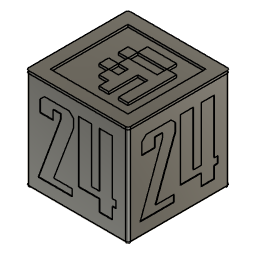
AutonOhm Apriltag 24 (Autodesk Fusion 360 design; units mm, degrees)
Autodesk Fusion 360 part; units mm, degrees
sketch "Skizze1" plane through (0, 0, 0) normal (0, 0, 1) x (1, 0, 0)
  line L0 (21, -21) -> (-21, -21)
  line L1 (-21, -21) -> (-21, 21)
  line L2 (-21, 21) -> (21, 21)
  line L3 (21, 21) -> (21, -21)
  line L4 (21, -21) -> (-21, 21) construction
  line L5 (-21, -21) -> (21, 21) construction
  dimension "d1" = 42
  dimension "d2" = 42
  constraint horizontal L0
  constraint perpendicular L0 L1
  constraint parallel L0 L2
  constraint parallel L1 L3
  constraint coincident L4 origin
  constraint coincident L5 origin
  measures "d1" distance of L1.end L2.end
  measures "d2" distance of L0.end L1.end
extrude "Extrusion1" add sketch "Skizze1" along normal blind 41 makes body 1
sketch "Skizze2" plane through (0, 0, 41) normal (0, 0, 1) x (-1, 0, 0)
  line L0 (-21, -21) -> (21, -21)
  line L1 (21, -21) -> (21, 21)
  line L2 (21, 21) -> (-21, 21)
  line L3 (-21, 21) -> (-21, -21)
  line L4 (21, -21) -> (-21, -21)
  line L5 (-21, -21) -> (-21, 21)
  line L6 (-21, 21) -> (21, 21)
  line L7 (21, 21) -> (21, -21)
  line L8 (-16, 16) -> (16, 16)
  line L9 (16, 16) -> (16, -16)
  line L10 (16, -16) -> (-16, -16)
  line L11 (-16, -16) -> (-16, 16)
  line L12 (-16, 16) -> (16, -16) construction
  line L13 (16, 16) -> (-16, -16) construction
  dimension "d5" = 32
  dimension "d6" = 32
  constraint horizontal L4
  constraint vertical L5
  constraint horizontal L6
  constraint vertical L7
  constraint coincident L2.end L3.start
  constraint coincident L0.end L1.start
  constraint horizontal L8
  constraint perpendicular L8 L9
  constraint parallel L8 L10
  constraint parallel L9 L11
  constraint coincident L12 origin
  constraint coincident L13 origin
  measures "d5" distance of L9.end L10.end
  measures "d6" distance of L8.end L9.end
extrude "Extrusion2" add sketch "Skizze2" along normal blind 1 separate body makes body 2
fillet "Abrundung1" radius 1 8 edges at (-21, 21, 20.5) (-21, -21, 20.5) (-21, 0, 0) (0, -21, 0) (21, -21, 20.5) (21, 0, 0) (21, 21, 20.5) (0, 21, 0) on bodies 1
fillet "Abrundung2" radius 1 1 edges at (21, 21, 41.5) on bodies 2
fillet "Abrundung3" radius 1 1 edges at (21, -21, 41.5) on bodies 2
fillet "Abrundung4" radius 1 1 edges at (-21, -21, 41.5) on bodies 2
fillet "Abrundung5" radius 1 1 edges at (-21, 21, 41.5) on bodies 2
sketch "Skizze3" plane through (0, 0, 0) normal (0, 0, -1) x (1, 0, 0)
  line L0 (-20, -20) -> (20, -20)
  line L1 (20, -20) -> (20, 20)
  line L2 (20, 20) -> (-20, 20)
  line L3 (-20, 20) -> (-20, -20)
  line L4 (-15.5554, -7.5319) -> (-15.5554, -12.9394)
  line L5 (-15.5554, -12.9394) -> (-1.7653, -13.0619)
  line L6 (-1.7653, -13.0619) -> (-1.8353, -7.8468)
  spline S0 degree 3 poles (-1.8353, -7.8468) (-9.4573, -5.9337) (-9.4543, 8.1703) (-0.2245, 8.2733) knots 0 0 0 0 1 1 1 1
  spline S1 degree 3 poles (-0.2245, 8.2733) (9.1628, 8.378) (10.5465, -5.8261) (1.9583, -7.8813) knots 0 0 0 0 1 1 1 1
  line L7 (1.9583, -7.8813) -> (1.9723, -13.0334)
  spline S2 degree 3 poles (1.9723, -13.0334) (15.5516, -12.9722) (18.9797, 12.8679) (-0.1523, 13.061) knots 0 0 0 0 1 1 1 1
  spline S3 degree 3 poles (-0.1523, 13.061) (-11.1806, 13.1724) (-15.9327, 2.2058) (-10.2013, -7.6521) knots 0 0 0 0 1 1 1 1
  line L8 (-10.2013, -7.6521) -> (-15.5554, -7.5319)
extrude "Extrusion3" add sketch "Skizze3" against normal blind 0.6 separate body contours L4 L5 L6 S0 S1 L7 S2 S3 L8 makes body 3
sketch "Skizze4" plane through (0, 0, 41) normal (0, 0, 1) x (-1, 0, 0)
  arc A0 (21, 20) -> (20, 21) centre (20, 20) ccw
  line L0 (20, 21) -> (-20, 21)
  arc A1 (-20, 21) -> (-21, 20) centre (-20, 20) ccw
  line L1 (-21, 20) -> (-21, -20)
  arc A2 (-21, -20) -> (-20, -21) centre (-20, -20) ccw
  line L2 (-20, -21) -> (20, -21)
  arc A3 (20, -21) -> (21, -20) centre (20, -20) ccw
  line L3 (21, -20) -> (21, 20)
  line L4 (-19.9999, 19.9999) -> (20.0001, 19.9999)
  line L5 (20.0001, 19.9999) -> (20.0001, -20.0001)
  line L6 (20.0001, -20.0001) -> (-19.9999, -20.0001)
  line L7 (-19.9999, -20.0001) -> (-19.9999, 19.9999)
  line L8 (21, 21) -> (-21, 21)
  line L9 (-21, 21) -> (-21, -21)
  line L10 (-21, -21) -> (21, -21)
  line L11 (21, -21) -> (21, 21)
  line L12 (20.0001, 19.9999) -> (-19.9999, 19.9999)
  line L13 (-19.9999, 19.9999) -> (-19.9999, -20.0001)
  line L14 (-19.9999, -20.0001) -> (20.0001, -20.0001)
  line L15 (20.0001, -20.0001) -> (20.0001, 19.9999)
  line L16 (-12.038, 11.9999) -> (-12.038, -7.9999)
  line L17 (-12.038, -7.9999) -> (-8.0381, -7.9999)
  line L18 (-8.0381, -7.9999) -> (-8.0381, -11.9999)
  line L19 (-8.0381, -11.9999) -> (3.9619, -11.9999)
  line L20 (3.9619, -11.9999) -> (3.9619, -7.9999)
  line L21 (3.9619, -7.9999) -> (7.9621, -7.9999)
  line L22 (7.9621, -7.9999) -> (7.9621, -4)
  line L23 (7.9621, -4) -> (3.9619, -4)
  line L24 (3.9619, -4) -> (3.9619, 0)
  line L25 (3.9619, 0) -> (7.9621, 0)
  line L26 (7.9621, 0) -> (7.9621, 4)
  line L27 (7.9621, 4) -> (3.9619, 4)
  line L28 (3.9619, 4) -> (3.9619, 8)
  line L29 (3.9619, 8) -> (-0.0381, 8)
  line L30 (-0.0381, 8) -> (-0.0381, 11.9999)
  line L31 (-0.0381, 11.9999) -> (-4.0381, 11.9999)
  line L32 (-4.0381, 11.9999) -> (-4.0381, 0)
  line L33 (-4.0381, 0) -> (-8.0381, 0)
  line L34 (-8.0381, 0) -> (-8.0381, 11.9999)
  line L35 (-8.0381, 11.9999) -> (-12.038, 11.9999)
  line L36 (-0.0381, 4) -> (-0.0381, 0)
  line L37 (-0.0381, 0) -> (3.9619, 0)
  line L38 (3.9619, 0) -> (3.9619, 4)
  line L39 (3.9619, 4) -> (-0.0381, 4)
  line L40 (-8.0381, -3.9999) -> (-8.0381, -7.9999)
  line L41 (-8.0381, -7.9999) -> (3.9619, -7.9999)
  line L42 (3.9619, -7.9999) -> (3.9619, -4)
  line L43 (3.9619, -4) -> (-8.0381, -3.9999)
extrude "Extrusion4" add sketch "Skizze4" along normal blind 1 separate body contours L16 L17 L24 L28 L29 L30 L31 L32 L33 L34 L35 L36 L37 L39 L40 L43 | L18 L19 L20 L41 | L21 L22 L23 L42 | L25 L26 L27 L38 makes body 4 at (10.7047, -1.3333, 41)
sketch "Skizze5" plane through (0, -21, 0) normal (0, -1, 0) x (1, 0, 0)
  line L0 (-20, 41) -> (-20, 1)
  line L1 (-20, 1) -> (20, 1)
  line L2 (20, 1) -> (20, 41)
  line L3 (20, 41) -> (-20, 41)
  line L4 (21, 42) -> (-21, 42)
  line L5 (-21, 42) -> (-21, 0)
  line L6 (-21, 0) -> (21, 0)
  line L7 (21, 0) -> (21, 42)
  line L8 (20.0001, 40.9999) -> (-19.9999, 40.9999)
  line L9 (-19.9999, 40.9999) -> (-19.9999, 0.9999)
  line L10 (-19.9999, 0.9999) -> (20.0001, 0.9999)
  line L11 (20.0001, 0.9999) -> (20.0001, 40.9999)
  line L12 (21, 0) -> (21, 6)
  line L13 (21, 6) -> (-21, 6)
  line L14 (-21, 6) -> (-21, 0)
  line L15 (-21, 0) -> (21, 0)
  line L16 (-21, 42) -> (-21, 36)
  line L17 (-21, 36) -> (21, 36)
  line L18 (21, 36) -> (21, 42)
  line L19 (21, 42) -> (-21, 42)
  line L20 (-1.4179, 34.153) -> (-3.2274, 35.9625)
  line L21 (-3.2274, 35.9625) -> (-13.4454, 35.9625)
  line L22 (-13.4454, 35.9625) -> (-15.2903, 34.153)
  line L23 (-15.2903, 34.153) -> (-15.2903, 29.3278)
  line L24 (-15.2903, 29.3278) -> (-9.8621, 29.3278)
  line L25 (-9.8621, 29.3278) -> (-9.8621, 33.124)
  line L26 (-9.8621, 33.124) -> (-6.7752, 33.124)
  line L27 (-6.7752, 33.124) -> (-6.7752, 31.2082)
  line L28 (-6.7752, 31.2082) -> (-15.9999, 5.9823)
  line L29 (-15.9999, 5.9823) -> (-2.0209, 5.9823)
  line L30 (-2.0209, 5.9823) -> (-2.0209, 8.8205)
  line L31 (-2.0209, 8.8205) -> (-9.6137, 8.8205)
  line L32 (-9.6137, 8.8205) -> (-1.4179, 30.747)
  line L33 (-1.4179, 30.747) -> (-1.4179, 34.153)
  line L34 (16.0382, 13.5748) -> (14.5481, 13.5748)
  line L35 (14.5481, 13.5748) -> (14.5481, 35.9625)
  line L36 (14.5481, 35.9625) -> (9.1905, 35.9625)
  line L37 (9.1905, 35.9625) -> (9.1905, 13.5748)
  line L38 (9.1905, 13.5748) -> (5.9618, 13.5748)
  line L39 (5.9618, 13.5748) -> (5.9618, 35.9625)
  line L40 (5.9618, 35.9625) -> (0.6045, 35.9625)
  line L41 (0.6045, 35.9625) -> (0.6045, 10.772)
  line L42 (0.6045, 10.772) -> (9.1905, 10.772)
  line L43 (9.1905, 10.772) -> (9.1905, 5.9823)
  line L44 (9.1905, 5.9823) -> (14.5481, 5.9823)
  line L45 (14.5481, 5.9823) -> (14.5481, 10.772)
  line L46 (14.5481, 10.772) -> (16.0382, 10.772)
  line L47 (16.0382, 10.772) -> (16.0382, 13.5748)
extrude "Extrusion5" cut sketch "Skizze5" against normal blind 0.2 contours L13 L20 L21 L22 L23 L24 L25 L26 L27 L28 L30 L31 L32 L33 | L13 L34 L35 L36 L37 L38 L39 L40 L41 L42 L43 L45 L46 L47 bodies 1
sketch "Skizze6" plane through (-21, 0, 0) normal (-1, 0, 0) x (0, -1, 0)
  line L0 (20, 1) -> (20, 41)
  line L1 (20, 41) -> (-20, 41)
  line L2 (-20, 41) -> (-20, 1)
  line L3 (-20, 1) -> (20, 1)
  line L4 (21, 42) -> (-21, 42)
  line L5 (-21, 42) -> (-21, 0)
  line L6 (-21, 0) -> (21, 0)
  line L7 (21, 0) -> (21, 42)
  line L8 (20.0001, 40.9999) -> (-19.9999, 40.9999)
  line L9 (-19.9999, 40.9999) -> (-19.9999, 0.9999)
  line L10 (-19.9999, 0.9999) -> (20.0001, 0.9999)
  line L11 (20.0001, 0.9999) -> (20.0001, 40.9999)
  line L12 (21, 0) -> (21, 6)
  line L13 (21, 6) -> (-21, 6)
  line L14 (-21, 6) -> (-21, 0)
  line L15 (-21, 0) -> (21, 0)
  line L16 (-21, 42) -> (-21, 36)
  line L17 (-21, 36) -> (21, 36)
  line L18 (21, 36) -> (21, 42)
  line L19 (21, 42) -> (-21, 42)
  line L20 (-1.4179, 34.153) -> (-3.2274, 35.9625)
  line L21 (-3.2274, 35.9625) -> (-13.4454, 35.9625)
  line L22 (-13.4454, 35.9625) -> (-15.2903, 34.153)
  line L23 (-15.2903, 34.153) -> (-15.2903, 29.3278)
  line L24 (-15.2903, 29.3278) -> (-9.8621, 29.3278)
  line L25 (-9.8621, 29.3278) -> (-9.8621, 33.124)
  line L26 (-9.8621, 33.124) -> (-6.7752, 33.124)
  line L27 (-6.7752, 33.124) -> (-6.7752, 31.2082)
  line L28 (-6.7752, 31.2082) -> (-15.9999, 5.9823)
  line L29 (-15.9999, 5.9823) -> (-2.0209, 5.9823)
  line L30 (-2.0209, 5.9823) -> (-2.0209, 8.8205)
  line L31 (-2.0209, 8.8205) -> (-9.6137, 8.8205)
  line L32 (-9.6137, 8.8205) -> (-1.4179, 30.747)
  line L33 (-1.4179, 30.747) -> (-1.4179, 34.153)
  line L34 (16.0382, 13.5748) -> (14.5481, 13.5748)
  line L35 (14.5481, 13.5748) -> (14.5481, 35.9625)
  line L36 (14.5481, 35.9625) -> (9.1905, 35.9625)
  line L37 (9.1905, 35.9625) -> (9.1905, 13.5748)
  line L38 (9.1905, 13.5748) -> (5.9618, 13.5748)
  line L39 (5.9618, 13.5748) -> (5.9618, 35.9625)
  line L40 (5.9618, 35.9625) -> (0.6045, 35.9625)
  line L41 (0.6045, 35.9625) -> (0.6045, 10.772)
  line L42 (0.6045, 10.772) -> (9.1905, 10.772)
  line L43 (9.1905, 10.772) -> (9.1905, 5.9823)
  line L44 (9.1905, 5.9823) -> (14.5481, 5.9823)
  line L45 (14.5481, 5.9823) -> (14.5481, 10.772)
  line L46 (14.5481, 10.772) -> (16.0382, 10.772)
  line L47 (16.0382, 10.772) -> (16.0382, 13.5748)
extrude "Extrusion6" cut sketch "Skizze6" against normal blind 0.2 contours L13 L34 L35 L36 L37 L38 L39 L40 L41 L42 L43 L45 L46 L47 | L13 L20 L21 L22 L23 L24 L25 L26 L27 L28 L30 L31 L32 L33 bodies 1
sketch "Skizze7" plane through (0, 21, 0) normal (0, 1, 0) x (-1, 0, 0)
  line L0 (20, 1) -> (20, 41)
  line L1 (20, 41) -> (-20, 41)
  line L2 (-20, 41) -> (-20, 1)
  line L3 (-20, 1) -> (20, 1)
  line L4 (21, 42) -> (-21, 42)
  line L5 (-21, 42) -> (-21, 0)
  line L6 (-21, 0) -> (21, 0)
  line L7 (21, 0) -> (21, 42)
  line L8 (20.0001, 40.9999) -> (-19.9999, 40.9999)
  line L9 (-19.9999, 40.9999) -> (-19.9999, 0.9999)
  line L10 (-19.9999, 0.9999) -> (20.0001, 0.9999)
  line L11 (20.0001, 0.9999) -> (20.0001, 40.9999)
  line L12 (21, 0) -> (21, 6)
  line L13 (21, 6) -> (-21, 6)
  line L14 (-21, 6) -> (-21, 0)
  line L15 (-21, 0) -> (21, 0)
  line L16 (-21, 42) -> (-21, 36)
  line L17 (-21, 36) -> (21, 36)
  line L18 (21, 36) -> (21, 42)
  line L19 (21, 42) -> (-21, 42)
  line L20 (-1.4179, 34.153) -> (-3.2274, 35.9625)
  line L21 (-3.2274, 35.9625) -> (-13.4454, 35.9625)
  line L22 (-13.4454, 35.9625) -> (-15.2903, 34.153)
  line L23 (-15.2903, 34.153) -> (-15.2903, 29.3278)
  line L24 (-15.2903, 29.3278) -> (-9.8621, 29.3278)
  line L25 (-9.8621, 29.3278) -> (-9.8621, 33.124)
  line L26 (-9.8621, 33.124) -> (-6.7752, 33.124)
  line L27 (-6.7752, 33.124) -> (-6.7752, 31.2082)
  line L28 (-6.7752, 31.2082) -> (-15.9999, 5.9823)
  line L29 (-15.9999, 5.9823) -> (-2.0209, 5.9823)
  line L30 (-2.0209, 5.9823) -> (-2.0209, 8.8205)
  line L31 (-2.0209, 8.8205) -> (-9.6137, 8.8205)
  line L32 (-9.6137, 8.8205) -> (-1.4179, 30.747)
  line L33 (-1.4179, 30.747) -> (-1.4179, 34.153)
  line L34 (16.0382, 13.5748) -> (14.5481, 13.5748)
  line L35 (14.5481, 13.5748) -> (14.5481, 35.9625)
  line L36 (14.5481, 35.9625) -> (9.1905, 35.9625)
  line L37 (9.1905, 35.9625) -> (9.1905, 13.5748)
  line L38 (9.1905, 13.5748) -> (5.9618, 13.5748)
  line L39 (5.9618, 13.5748) -> (5.9618, 35.9625)
  line L40 (5.9618, 35.9625) -> (0.6045, 35.9625)
  line L41 (0.6045, 35.9625) -> (0.6045, 10.772)
  line L42 (0.6045, 10.772) -> (9.1905, 10.772)
  line L43 (9.1905, 10.772) -> (9.1905, 5.9823)
  line L44 (9.1905, 5.9823) -> (14.5481, 5.9823)
  line L45 (14.5481, 5.9823) -> (14.5481, 10.772)
  line L46 (14.5481, 10.772) -> (16.0382, 10.772)
  line L47 (16.0382, 10.772) -> (16.0382, 13.5748)
extrude "Extrusion7" cut sketch "Skizze7" against normal blind 0.2 contours L13 L34 L35 L36 L37 L38 L39 L40 L41 L42 L43 L45 L46 L47 | L13 L20 L21 L22 L23 L24 L25 L26 L27 L28 L30 L31 L32 L33 bodies 1
sketch "Skizze8" plane through (21, 0, 0) normal (1, 0, 0) x (0, 1, 0)
  line L0 (-20, 41) -> (-20, 1)
  line L1 (-20, 1) -> (20, 1)
  line L2 (20, 1) -> (20, 41)
  line L3 (20, 41) -> (-20, 41)
  line L4 (21, 42) -> (-21, 42)
  line L5 (-21, 42) -> (-21, 0)
  line L6 (-21, 0) -> (21, 0)
  line L7 (21, 0) -> (21, 42)
  line L8 (20.0001, 40.9999) -> (-19.9999, 40.9999)
  line L9 (-19.9999, 40.9999) -> (-19.9999, 0.9999)
  line L10 (-19.9999, 0.9999) -> (20.0001, 0.9999)
  line L11 (20.0001, 0.9999) -> (20.0001, 40.9999)
  line L12 (21, 0) -> (21, 6)
  line L13 (21, 6) -> (-21, 6)
  line L14 (-21, 6) -> (-21, 0)
  line L15 (-21, 0) -> (21, 0)
  line L16 (-21, 42) -> (-21, 36)
  line L17 (-21, 36) -> (21, 36)
  line L18 (21, 36) -> (21, 42)
  line L19 (21, 42) -> (-21, 42)
  line L20 (-1.4179, 34.153) -> (-3.2274, 35.9625)
  line L21 (-3.2274, 35.9625) -> (-13.4454, 35.9625)
  line L22 (-13.4454, 35.9625) -> (-15.2903, 34.153)
  line L23 (-15.2903, 34.153) -> (-15.2903, 29.3278)
  line L24 (-15.2903, 29.3278) -> (-9.8621, 29.3278)
  line L25 (-9.8621, 29.3278) -> (-9.8621, 33.124)
  line L26 (-9.8621, 33.124) -> (-6.7752, 33.124)
  line L27 (-6.7752, 33.124) -> (-6.7752, 31.2082)
  line L28 (-6.7752, 31.2082) -> (-15.9999, 5.9823)
  line L29 (-15.9999, 5.9823) -> (-2.0209, 5.9823)
  line L30 (-2.0209, 5.9823) -> (-2.0209, 8.8205)
  line L31 (-2.0209, 8.8205) -> (-9.6137, 8.8205)
  line L32 (-9.6137, 8.8205) -> (-1.4179, 30.747)
  line L33 (-1.4179, 30.747) -> (-1.4179, 34.153)
  line L34 (16.0382, 13.5748) -> (14.5481, 13.5748)
  line L35 (14.5481, 13.5748) -> (14.5481, 35.9625)
  line L36 (14.5481, 35.9625) -> (9.1905, 35.9625)
  line L37 (9.1905, 35.9625) -> (9.1905, 13.5748)
  line L38 (9.1905, 13.5748) -> (5.9618, 13.5748)
  line L39 (5.9618, 13.5748) -> (5.9618, 35.9625)
  line L40 (5.9618, 35.9625) -> (0.6045, 35.9625)
  line L41 (0.6045, 35.9625) -> (0.6045, 10.772)
  line L42 (0.6045, 10.772) -> (9.1905, 10.772)
  line L43 (9.1905, 10.772) -> (9.1905, 5.9823)
  line L44 (9.1905, 5.9823) -> (14.5481, 5.9823)
  line L45 (14.5481, 5.9823) -> (14.5481, 10.772)
  line L46 (14.5481, 10.772) -> (16.0382, 10.772)
  line L47 (16.0382, 10.772) -> (16.0382, 13.5748)
extrude "Extrusion8" cut sketch "Skizze8" against normal blind 0.2 contours L13 L20 L21 L22 L23 L24 L25 L26 L27 L28 L30 L31 L32 L33 | L13 L34 L35 L36 L37 L38 L39 L40 L41 L42 L43 L45 L46 L47 bodies 1
named bodies: "Grundkörper", "Apriltag Kranz", "OhmLogo Unterseite"
